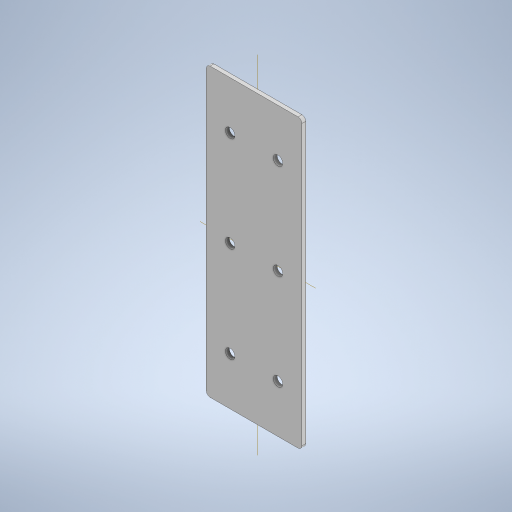
# Autodesk Inventor part: joint
Saved by Autodesk Inventor 2024 (Build 280153000, 153)
## iProperties
Created: 2024-02-27
Part Number: joint
Material: Generic
Document SubType Name: Modeling
Designer: Administrator
Density: 1 g/cm^3
Appearance: Default
Author: Administrator
Autodesk Inventor part; units mm, degrees
ref_plane "YZ Plane" through (0, 0, 0) normal (1, 0, 0) x (0, 1, 0)
ref_plane "XZ Plane" through (0, 0, 0) normal (0, 1, 0) x (-1, 0, 0)
ref_plane "XY Plane" through (0, 0, 0) normal (0, 0, 1) x (1, 0, 0)
sketch "Sketch1" plane through (0, 0, 0) normal (0, 0, 1) x (1, 0, 0)
  line L0 (-23, 75) -> (23, 75)
  line L1 (25, 73) -> (25, -73)
  line L2 (23, -75) -> (-23, -75)
  line L3 (-25, -73) -> (-25, 73)
  arc A0 (-23, 75) -> (-25, 73) centre (-23, 73) ccw
  arc A1 (25, 73) -> (23, 75) centre (23, 73) ccw
  arc A2 (23, -75) -> (25, -73) centre (23, -73) ccw
  arc A3 (-25, -73) -> (-23, -75) centre (-23, -73) ccw
  point P0 (0, 0)
  point P1 (-25, 75)
  point P2 (25, 75)
  point P3 (-25, -75)
  point P4 (-25, 0)
  dimension "d0" = 50
  dimension "d1" = 150
  dimension "d2" = 25
  dimension "d3" = 75
  dimension "d4" = 2
  dimension "d5" = 2
  dimension "d6" = 2
  dimension "d7" = 2
  constraints: 8 end point, 8 point on circle, 8 tangent, 6 point on line, 4 centre point, 2 parallel, 1 horizontal, 1 midpoint, 1 perpendicular
  measures "d0" distance of point (-25, 75) point (25, 75)
  measures "d1" distance of point (-25, -75) point (-25, 75)
  measures "d2" distance of point (0, 0) point (-25, 0)
  measures "d3" distance from line of point (0, 0) L0
  measures "d4" radius of A0
  measures "d5" radius of A1
  measures "d6" radius of A2
  measures "d7" radius of A3
extrude "Extrusion1" add sketch "Sketch1" along normal blind 2
sketch "Sketch2" plane through (0, 0, 2) normal (0, 0, 1) x (1, 0, 0)
  line L0 (-64, 0) -> (59, 0)
  line L1 (0, 89) -> (0, -64)
  line L2 (-25, 73) -> (-25, -73) projected
  line L3 (23, 75) -> (-23, 75) projected
  point P0 (0, 0)
  point P1 (-12.5, 50)
  point P2 (-12.5, 0)
  point P3 (-12.5, -50)
  point P4 (12.5, 50)
  point P5 (12.5, 0)
  point P6 (12.5, -50)
  dimension "d12" = 50
  dimension "d15" = 25
  dimension "d18" = 12.5
  dimension "d19" = 25
  constraints: 4 end point, 2 horizontal, 2 vertical, 5 other
  measures "d12" distance of point (-12.5, 50) point (-12.5, 0)
  measures "d15" distance of point (-12.5, 50) point (12.5, 50)
  measures "d18" distance from line of L2 point (-12.5, 50)
  measures "d19" distance from line of L3 point (-12.5, 50)
hole "Hole1" at (-12.5, 50, 2) at (-12.5, 0, 2) at (-12.5, -50, 2) at (12.5, 50, 2) at (12.5, 0, 2) at (12.5, -50, 2) direction (0, 0, -1) diameter 5 end through all
body "Solid1"
